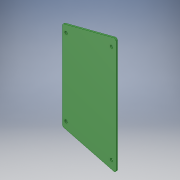
# Autodesk Inventor part: PCBCapteurs
Saved by Autodesk Inventor 2019 (Build 230136000, 136)
## iProperties
Created: 2019-07-30
Part Number: PCBCapteurs
Material: Résine phénolique
Document SubType Name: Modeling
Designer: Sébastien DI MERCURIO
Mass: 15.8976 g
Surface Area: 149.76 cm^2
Volume: 11.52 cm^3
Density: 1.38 g/cm^3
Appearance: Lisse - Vert forêt foncé
Author: Sébastien DI MERCURIO
Autodesk Inventor part; units mm, degrees
ref_plane "YZ Plane" through (0, 0, 0) normal (1, 0, 0) x (0, 1, 0)
ref_plane "XZ Plane" through (0, 0, 0) normal (0, 1, 0) x (-1, 0, 0)
ref_plane "XY Plane" through (0, 0, 0) normal (0, 0, 1) x (1, 0, 0)
sketch "Esquisse1" plane through (0, 0, 0) normal (0, 0, 1) x (1, 0, 0)
  line L0 (0, 0) -> (60, 0)
  line L1 (60, 0) -> (60, 130)
  line L2 (60, 130) -> (0, 130)
  line L3 (0, 130) -> (0, 0)
  dimension "d0" = 130
  dimension "d1" = 60
  constraints: 8 end point, 2 parallel, 1 horizontal, 1 perpendicular
  measures "d0" distance of L2.end L0.start
  measures "d1" distance of L1.end L2.end
extrude "Extrusion1" add sketch "Esquisse1" along normal blind 1.6
chamfer "Chanfrein1" distance 58 distance2 15 1 edges at (0, 130, 0.8) measured on face at (40, 130, 0.5333)
chamfer "Chanfrein2" distance 15 distance2 58 1 edges at (0, 0, 0.8) measured on face at (0, 76.6667, 1.0667)
fillet "Congé1" radius 2 6 edges at (60, 0, 0.8) (0, 15, 0.8) (0, 115, 0.8) (60, 130, 0.8) (58, 130, 0.8) (58, 0, 0.8)
sketch "Esquisse2" plane through (0, 0, 1.6) normal (0, 0, 1) x (1, 0, 0)
  circle A0 centre (4, 22) radius 1.6
  circle A1 centre (55, 10) radius 1.6
  circle A2 centre (4, 108) radius 1.6
  circle A3 centre (55, 120) radius 1.6
  line L0 (0, 113.4514) -> (0, 16.5486) projected
  arc A4 (57.4992, 0.1295) -> (60, 2.0658) centre (58, 2.0658) ccw projected
  arc A5 (60, 127.9342) -> (57.4992, 129.8705) centre (58, 127.9342) ccw projected
  point P0 (0, 0)
  dimension "d11" = 51
  dimension "d12" = 4
  dimension "d13" = 86
  dimension "d14" = 96.9029
  dimension "d15" = 5.4514
  dimension "d16" = 110
  dimension "d17" = 125.8684
  dimension "d18" = 7.9342
  dimension "d19" = 3.2
  constraints: 4 centre point, 3 equal radius, 2 vertical alignment
  measures "d11" horizontal distance of A3.centre A2.centre
  measures "d12" distance from line of L0 A2.centre
  measures "d13" distance of A0.centre A2.centre
  measures "d14" distance of L0.end L0.start
  measures "d15" vertical distance of L0.start A2.centre
  measures "d16" distance of A1.centre A3.centre
  measures "d17" distance of A4.centre A5.centre
  measures "d18" vertical distance of A4.centre A1.centre
  measures "d19" diameter of A1
extrude "Extrusion2" cut sketch "Esquisse2" against normal through all
equation "\"d15\" = -0.5 * d13 + 0.5 * d14"
equation "\"d18\" = -0.5 * d16 + 0.5 * d17"
